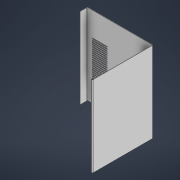
# Autodesk Inventor part: PlateAMP
Saved by Autodesk Inventor 2022 (Build 260153070, 153G)
## iProperties
Created: 2021-12-15
Part Number: PlateAMP
Material: Типовые
Document SubType Name: Sheet Metal
Designer: kalugin_a
Density: 1 g/cm^3
Flat Pattern Width: 26.5 cm
Flat Pattern Length: 43.9179 cm
Flat Pattern Area: 1163.82 cm^2
Sheet Metal Rule: По умолчанию_мм
Sheet Metal Width: 265,000 мм
Sheet Metal Length: 439,179 мм
Sheet Metal Area: 116382,371 мм^2
Appearance: По умолчанию
Author: kalugin_a
Autodesk Inventor part; units mm, degrees
ref_plane "YZ Plane" through (0, 0, 0) normal (1, 0, 0) x (0, 1, 0)
ref_plane "XZ Plane" through (0, 0, 0) normal (0, 1, 0) x (-1, 0, 0)
ref_plane "XY Plane" through (0, 0, 0) normal (0, 0, 1) x (1, 0, 0)
sketch "Эскиз1" plane through (0, 0, 0) normal (0, 0, 1) x (1, 0, 0)
  line L0 (0, 0) -> (217, 0)
  line L1 (217, 0) -> (217, 265)
  line L2 (217, 265) -> (0, 265)
  line L3 (0, 265) -> (0, 0)
  line L4 (207.9674, 23.6384) -> (147.9674, 23.6384) construction
  line L5 (206.4674, 25.1384) -> (149.4674, 25.1384)
  line L6 (149.4674, 22.1384) -> (206.4674, 22.1384)
  arc A0 (206.4674, 22.1384) -> (206.4674, 25.1384) centre (206.4674, 23.6384) ccw
  arc A1 (149.4674, 25.1384) -> (149.4674, 22.1384) centre (149.4674, 23.6384) ccw
  line L7 (207.9674, 29.6384) -> (147.9674, 29.6384) construction
  line L8 (206.4674, 31.1384) -> (149.4674, 31.1384)
  line L9 (149.4674, 28.1384) -> (206.4674, 28.1384)
  arc A2 (206.4674, 28.1384) -> (206.4674, 31.1384) centre (206.4674, 29.6384) ccw
  arc A3 (149.4674, 31.1384) -> (149.4674, 28.1384) centre (149.4674, 29.6384) ccw
  line L10 (207.9674, 35.6384) -> (147.9674, 35.6384) construction
  line L11 (206.4674, 37.1384) -> (149.4674, 37.1384)
  line L12 (149.4674, 34.1384) -> (206.4674, 34.1384)
  arc A4 (206.4674, 34.1384) -> (206.4674, 37.1384) centre (206.4674, 35.6384) ccw
  arc A5 (149.4674, 37.1384) -> (149.4674, 34.1384) centre (149.4674, 35.6384) ccw
  line L13 (207.9674, 41.6384) -> (147.9674, 41.6384) construction
  line L14 (206.4674, 43.1384) -> (149.4674, 43.1384)
  line L15 (149.4674, 40.1384) -> (206.4674, 40.1384)
  arc A6 (206.4674, 40.1384) -> (206.4674, 43.1384) centre (206.4674, 41.6384) ccw
  arc A7 (149.4674, 43.1384) -> (149.4674, 40.1384) centre (149.4674, 41.6384) ccw
  line L16 (207.9674, 47.6384) -> (147.9674, 47.6384) construction
  line L17 (206.4674, 49.1384) -> (149.4674, 49.1384)
  line L18 (149.4674, 46.1384) -> (206.4674, 46.1384)
  arc A8 (206.4674, 46.1384) -> (206.4674, 49.1384) centre (206.4674, 47.6384) ccw
  arc A9 (149.4674, 49.1384) -> (149.4674, 46.1384) centre (149.4674, 47.6384) ccw
  line L19 (207.9674, 53.6384) -> (147.9674, 53.6384) construction
  line L20 (206.4674, 55.1384) -> (149.4674, 55.1384)
  line L21 (149.4674, 52.1384) -> (206.4674, 52.1384)
  arc A10 (206.4674, 52.1384) -> (206.4674, 55.1384) centre (206.4674, 53.6384) ccw
  arc A11 (149.4674, 55.1384) -> (149.4674, 52.1384) centre (149.4674, 53.6384) ccw
  line L22 (207.9674, 59.6384) -> (147.9674, 59.6384) construction
  line L23 (206.4674, 61.1384) -> (149.4674, 61.1384)
  line L24 (149.4674, 58.1384) -> (206.4674, 58.1384)
  arc A12 (206.4674, 58.1384) -> (206.4674, 61.1384) centre (206.4674, 59.6384) ccw
  arc A13 (149.4674, 61.1384) -> (149.4674, 58.1384) centre (149.4674, 59.6384) ccw
  line L25 (207.9674, 65.6384) -> (147.9674, 65.6384) construction
  line L26 (206.4674, 67.1384) -> (149.4674, 67.1384)
  line L27 (149.4674, 64.1384) -> (206.4674, 64.1384)
  arc A14 (206.4674, 64.1384) -> (206.4674, 67.1384) centre (206.4674, 65.6384) ccw
  arc A15 (149.4674, 67.1384) -> (149.4674, 64.1384) centre (149.4674, 65.6384) ccw
  line L28 (207.9674, 71.6384) -> (147.9674, 71.6384) construction
  line L29 (206.4674, 73.1384) -> (149.4674, 73.1384)
  line L30 (149.4674, 70.1384) -> (206.4674, 70.1384)
  arc A16 (206.4674, 70.1384) -> (206.4674, 73.1384) centre (206.4674, 71.6384) ccw
  arc A17 (149.4674, 73.1384) -> (149.4674, 70.1384) centre (149.4674, 71.6384) ccw
  line L31 (207.9674, 77.6384) -> (147.9674, 77.6384) construction
  line L32 (206.4674, 79.1384) -> (149.4674, 79.1384)
  line L33 (149.4674, 76.1384) -> (206.4674, 76.1384)
  arc A18 (206.4674, 76.1384) -> (206.4674, 79.1384) centre (206.4674, 77.6384) ccw
  arc A19 (149.4674, 79.1384) -> (149.4674, 76.1384) centre (149.4674, 77.6384) ccw
  line L34 (207.9674, 83.6384) -> (147.9674, 83.6384) construction
  line L35 (206.4674, 85.1384) -> (149.4674, 85.1384)
  line L36 (149.4674, 82.1384) -> (206.4674, 82.1384)
  arc A20 (206.4674, 82.1384) -> (206.4674, 85.1384) centre (206.4674, 83.6384) ccw
  arc A21 (149.4674, 85.1384) -> (149.4674, 82.1384) centre (149.4674, 83.6384) ccw
  line L37 (207.9674, 89.6384) -> (147.9674, 89.6384) construction
  line L38 (206.4674, 91.1384) -> (149.4674, 91.1384)
  line L39 (149.4674, 88.1384) -> (206.4674, 88.1384)
  arc A22 (206.4674, 88.1384) -> (206.4674, 91.1384) centre (206.4674, 89.6384) ccw
  arc A23 (149.4674, 91.1384) -> (149.4674, 88.1384) centre (149.4674, 89.6384) ccw
  line L40 (207.9674, 95.6384) -> (147.9674, 95.6384) construction
  line L41 (206.4674, 97.1384) -> (149.4674, 97.1384)
  line L42 (149.4674, 94.1384) -> (206.4674, 94.1384)
  arc A24 (206.4674, 94.1384) -> (206.4674, 97.1384) centre (206.4674, 95.6384) ccw
  arc A25 (149.4674, 97.1384) -> (149.4674, 94.1384) centre (149.4674, 95.6384) ccw
  line L43 (207.9674, 101.6384) -> (147.9674, 101.6384) construction
  line L44 (206.4674, 103.1384) -> (149.4674, 103.1384)
  line L45 (149.4674, 100.1384) -> (206.4674, 100.1384)
  arc A26 (206.4674, 100.1384) -> (206.4674, 103.1384) centre (206.4674, 101.6384) ccw
  arc A27 (149.4674, 103.1384) -> (149.4674, 100.1384) centre (149.4674, 101.6384) ccw
  line L46 (207.9674, 107.6384) -> (147.9674, 107.6384) construction
  line L47 (206.4674, 109.1384) -> (149.4674, 109.1384)
  line L48 (149.4674, 106.1384) -> (206.4674, 106.1384)
  arc A28 (206.4674, 106.1384) -> (206.4674, 109.1384) centre (206.4674, 107.6384) ccw
  arc A29 (149.4674, 109.1384) -> (149.4674, 106.1384) centre (149.4674, 107.6384) ccw
  line L49 (207.9674, 113.6384) -> (147.9674, 113.6384) construction
  line L50 (206.4674, 115.1384) -> (149.4674, 115.1384)
  line L51 (149.4674, 112.1384) -> (206.4674, 112.1384)
  arc A30 (206.4674, 112.1384) -> (206.4674, 115.1384) centre (206.4674, 113.6384) ccw
  arc A31 (149.4674, 115.1384) -> (149.4674, 112.1384) centre (149.4674, 113.6384) ccw
  line L52 (207.9674, 119.6384) -> (147.9674, 119.6384) construction
  line L53 (206.4674, 121.1384) -> (149.4674, 121.1384)
  line L54 (149.4674, 118.1384) -> (206.4674, 118.1384)
  arc A32 (206.4674, 118.1384) -> (206.4674, 121.1384) centre (206.4674, 119.6384) ccw
  arc A33 (149.4674, 121.1384) -> (149.4674, 118.1384) centre (149.4674, 119.6384) ccw
  line L55 (207.9674, 125.6384) -> (147.9674, 125.6384) construction
  line L56 (206.4674, 127.1384) -> (149.4674, 127.1384)
  line L57 (149.4674, 124.1384) -> (206.4674, 124.1384)
  arc A34 (206.4674, 124.1384) -> (206.4674, 127.1384) centre (206.4674, 125.6384) ccw
  arc A35 (149.4674, 127.1384) -> (149.4674, 124.1384) centre (149.4674, 125.6384) ccw
  line L58 (207.9674, 131.6384) -> (147.9674, 131.6384) construction
  line L59 (206.4674, 133.1384) -> (149.4674, 133.1384)
  line L60 (149.4674, 130.1384) -> (206.4674, 130.1384)
  arc A36 (206.4674, 130.1384) -> (206.4674, 133.1384) centre (206.4674, 131.6384) ccw
  arc A37 (149.4674, 133.1384) -> (149.4674, 130.1384) centre (149.4674, 131.6384) ccw
  line L61 (207.9674, 137.6384) -> (147.9674, 137.6384) construction
  line L62 (206.4674, 139.1384) -> (149.4674, 139.1384)
  line L63 (149.4674, 136.1384) -> (206.4674, 136.1384)
  arc A38 (206.4674, 136.1384) -> (206.4674, 139.1384) centre (206.4674, 137.6384) ccw
  arc A39 (149.4674, 139.1384) -> (149.4674, 136.1384) centre (149.4674, 137.6384) ccw
  line L64 (207.9674, 143.6384) -> (147.9674, 143.6384) construction
  line L65 (206.4674, 145.1384) -> (149.4674, 145.1384)
  line L66 (149.4674, 142.1384) -> (206.4674, 142.1384)
  arc A40 (206.4674, 142.1384) -> (206.4674, 145.1384) centre (206.4674, 143.6384) ccw
  arc A41 (149.4674, 145.1384) -> (149.4674, 142.1384) centre (149.4674, 143.6384) ccw
  line L67 (207.9674, 149.6384) -> (147.9674, 149.6384) construction
  line L68 (206.4674, 151.1384) -> (149.4674, 151.1384)
  line L69 (149.4674, 148.1384) -> (206.4674, 148.1384)
  arc A42 (206.4674, 148.1384) -> (206.4674, 151.1384) centre (206.4674, 149.6384) ccw
  arc A43 (149.4674, 151.1384) -> (149.4674, 148.1384) centre (149.4674, 149.6384) ccw
  line L70 (207.9674, 155.6384) -> (147.9674, 155.6384) construction
  line L71 (206.4674, 157.1384) -> (149.4674, 157.1384)
  line L72 (149.4674, 154.1384) -> (206.4674, 154.1384)
  arc A44 (206.4674, 154.1384) -> (206.4674, 157.1384) centre (206.4674, 155.6384) ccw
  arc A45 (149.4674, 157.1384) -> (149.4674, 154.1384) centre (149.4674, 155.6384) ccw
  line L73 (207.9674, 161.6384) -> (147.9674, 161.6384) construction
  line L74 (206.4674, 163.1384) -> (149.4674, 163.1384)
  line L75 (149.4674, 160.1384) -> (206.4674, 160.1384)
  arc A46 (206.4674, 160.1384) -> (206.4674, 163.1384) centre (206.4674, 161.6384) ccw
  arc A47 (149.4674, 163.1384) -> (149.4674, 160.1384) centre (149.4674, 161.6384) ccw
  line L76 (77.9674, 23.6384) -> (17.9674, 23.6384) construction
  line L77 (76.4674, 25.1384) -> (19.4674, 25.1384)
  line L78 (19.4674, 22.1384) -> (76.4674, 22.1384)
  arc A48 (76.4674, 22.1384) -> (76.4674, 25.1384) centre (76.4674, 23.6384) ccw
  arc A49 (19.4674, 25.1384) -> (19.4674, 22.1384) centre (19.4674, 23.6384) ccw
  line L79 (77.9674, 29.6384) -> (17.9674, 29.6384) construction
  line L80 (76.4674, 31.1384) -> (19.4674, 31.1384)
  line L81 (19.4674, 28.1384) -> (76.4674, 28.1384)
  arc A50 (76.4674, 28.1384) -> (76.4674, 31.1384) centre (76.4674, 29.6384) ccw
  arc A51 (19.4674, 31.1384) -> (19.4674, 28.1384) centre (19.4674, 29.6384) ccw
  line L82 (77.9674, 35.6384) -> (17.9674, 35.6384) construction
  line L83 (76.4674, 37.1384) -> (19.4674, 37.1384)
  line L84 (19.4674, 34.1384) -> (76.4674, 34.1384)
  arc A52 (76.4674, 34.1384) -> (76.4674, 37.1384) centre (76.4674, 35.6384) ccw
  arc A53 (19.4674, 37.1384) -> (19.4674, 34.1384) centre (19.4674, 35.6384) ccw
  line L85 (77.9674, 41.6384) -> (17.9674, 41.6384) construction
  line L86 (76.4674, 43.1384) -> (19.4674, 43.1384)
  line L87 (19.4674, 40.1384) -> (76.4674, 40.1384)
  arc A54 (76.4674, 40.1384) -> (76.4674, 43.1384) centre (76.4674, 41.6384) ccw
  arc A55 (19.4674, 43.1384) -> (19.4674, 40.1384) centre (19.4674, 41.6384) ccw
  line L88 (77.9674, 47.6384) -> (17.9674, 47.6384) construction
  line L89 (76.4674, 49.1384) -> (19.4674, 49.1384)
  line L90 (19.4674, 46.1384) -> (76.4674, 46.1384)
  arc A56 (76.4674, 46.1384) -> (76.4674, 49.1384) centre (76.4674, 47.6384) ccw
  arc A57 (19.4674, 49.1384) -> (19.4674, 46.1384) centre (19.4674, 47.6384) ccw
  line L91 (77.9674, 53.6384) -> (17.9674, 53.6384) construction
  line L92 (76.4674, 55.1384) -> (19.4674, 55.1384)
  line L93 (19.4674, 52.1384) -> (76.4674, 52.1384)
  arc A58 (76.4674, 52.1384) -> (76.4674, 55.1384) centre (76.4674, 53.6384) ccw
  arc A59 (19.4674, 55.1384) -> (19.4674, 52.1384) centre (19.4674, 53.6384) ccw
  line L94 (77.9674, 59.6384) -> (17.9674, 59.6384) construction
  line L95 (76.4674, 61.1384) -> (19.4674, 61.1384)
  line L96 (19.4674, 58.1384) -> (76.4674, 58.1384)
  arc A60 (76.4674, 58.1384) -> (76.4674, 61.1384) centre (76.4674, 59.6384) ccw
  arc A61 (19.4674, 61.1384) -> (19.4674, 58.1384) centre (19.4674, 59.6384) ccw
  line L97 (77.9674, 65.6384) -> (17.9674, 65.6384) construction
  line L98 (76.4674, 67.1384) -> (19.4674, 67.1384)
  line L99 (19.4674, 64.1384) -> (76.4674, 64.1384)
  arc A62 (76.4674, 64.1384) -> (76.4674, 67.1384) centre (76.4674, 65.6384) ccw
  arc A63 (19.4674, 67.1384) -> (19.4674, 64.1384) centre (19.4674, 65.6384) ccw
  line L100 (77.9674, 71.6384) -> (17.9674, 71.6384) construction
  line L101 (76.4674, 73.1384) -> (19.4674, 73.1384)
  line L102 (19.4674, 70.1384) -> (76.4674, 70.1384)
  arc A64 (76.4674, 70.1384) -> (76.4674, 73.1384) centre (76.4674, 71.6384) ccw
  arc A65 (19.4674, 73.1384) -> (19.4674, 70.1384) centre (19.4674, 71.6384) ccw
  line L103 (77.9674, 77.6384) -> (17.9674, 77.6384) construction
  line L104 (76.4674, 79.1384) -> (19.4674, 79.1384)
  line L105 (19.4674, 76.1384) -> (76.4674, 76.1384)
  arc A66 (76.4674, 76.1384) -> (76.4674, 79.1384) centre (76.4674, 77.6384) ccw
  arc A67 (19.4674, 79.1384) -> (19.4674, 76.1384) centre (19.4674, 77.6384) ccw
  line L106 (77.9674, 83.6384) -> (17.9674, 83.6384) construction
  line L107 (76.4674, 85.1384) -> (19.4674, 85.1384)
  line L108 (19.4674, 82.1384) -> (76.4674, 82.1384)
  arc A68 (76.4674, 82.1384) -> (76.4674, 85.1384) centre (76.4674, 83.6384) ccw
  arc A69 (19.4674, 85.1384) -> (19.4674, 82.1384) centre (19.4674, 83.6384) ccw
  line L109 (77.9674, 89.6384) -> (17.9674, 89.6384) construction
  line L110 (76.4674, 91.1384) -> (19.4674, 91.1384)
  line L111 (19.4674, 88.1384) -> (76.4674, 88.1384)
  arc A70 (76.4674, 88.1384) -> (76.4674, 91.1384) centre (76.4674, 89.6384) ccw
  arc A71 (19.4674, 91.1384) -> (19.4674, 88.1384) centre (19.4674, 89.6384) ccw
  line L112 (77.9674, 95.6384) -> (17.9674, 95.6384) construction
  line L113 (76.4674, 97.1384) -> (19.4674, 97.1384)
  line L114 (19.4674, 94.1384) -> (76.4674, 94.1384)
  arc A72 (76.4674, 94.1384) -> (76.4674, 97.1384) centre (76.4674, 95.6384) ccw
  arc A73 (19.4674, 97.1384) -> (19.4674, 94.1384) centre (19.4674, 95.6384) ccw
  line L115 (77.9674, 101.6384) -> (17.9674, 101.6384) construction
  line L116 (76.4674, 103.1384) -> (19.4674, 103.1384)
  line L117 (19.4674, 100.1384) -> (76.4674, 100.1384)
  arc A74 (76.4674, 100.1384) -> (76.4674, 103.1384) centre (76.4674, 101.6384) ccw
  arc A75 (19.4674, 103.1384) -> (19.4674, 100.1384) centre (19.4674, 101.6384) ccw
  line L118 (77.9674, 107.6384) -> (17.9674, 107.6384) construction
  line L119 (76.4674, 109.1384) -> (19.4674, 109.1384)
  line L120 (19.4674, 106.1384) -> (76.4674, 106.1384)
  arc A76 (76.4674, 106.1384) -> (76.4674, 109.1384) centre (76.4674, 107.6384) ccw
  arc A77 (19.4674, 109.1384) -> (19.4674, 106.1384) centre (19.4674, 107.6384) ccw
  line L121 (77.9674, 113.6384) -> (17.9674, 113.6384) construction
  line L122 (76.4674, 115.1384) -> (19.4674, 115.1384)
  line L123 (19.4674, 112.1384) -> (76.4674, 112.1384)
  arc A78 (76.4674, 112.1384) -> (76.4674, 115.1384) centre (76.4674, 113.6384) ccw
  arc A79 (19.4674, 115.1384) -> (19.4674, 112.1384) centre (19.4674, 113.6384) ccw
  line L124 (77.9674, 119.6384) -> (17.9674, 119.6384) construction
  line L125 (76.4674, 121.1384) -> (19.4674, 121.1384)
  line L126 (19.4674, 118.1384) -> (76.4674, 118.1384)
  arc A80 (76.4674, 118.1384) -> (76.4674, 121.1384) centre (76.4674, 119.6384) ccw
  arc A81 (19.4674, 121.1384) -> (19.4674, 118.1384) centre (19.4674, 119.6384) ccw
  line L127 (77.9674, 125.6384) -> (17.9674, 125.6384) construction
  line L128 (76.4674, 127.1384) -> (19.4674, 127.1384)
  line L129 (19.4674, 124.1384) -> (76.4674, 124.1384)
  arc A82 (76.4674, 124.1384) -> (76.4674, 127.1384) centre (76.4674, 125.6384) ccw
  arc A83 (19.4674, 127.1384) -> (19.4674, 124.1384) centre (19.4674, 125.6384) ccw
  line L130 (77.9674, 131.6384) -> (17.9674, 131.6384) construction
  line L131 (76.4674, 133.1384) -> (19.4674, 133.1384)
  line L132 (19.4674, 130.1384) -> (76.4674, 130.1384)
  arc A84 (76.4674, 130.1384) -> (76.4674, 133.1384) centre (76.4674, 131.6384) ccw
  arc A85 (19.4674, 133.1384) -> (19.4674, 130.1384) centre (19.4674, 131.6384) ccw
  line L133 (77.9674, 137.6384) -> (17.9674, 137.6384) construction
  line L134 (76.4674, 139.1384) -> (19.4674, 139.1384)
  line L135 (19.4674, 136.1384) -> (76.4674, 136.1384)
  arc A86 (76.4674, 136.1384) -> (76.4674, 139.1384) centre (76.4674, 137.6384) ccw
  arc A87 (19.4674, 139.1384) -> (19.4674, 136.1384) centre (19.4674, 137.6384) ccw
  line L136 (77.9674, 143.6384) -> (17.9674, 143.6384) construction
  line L137 (76.4674, 145.1384) -> (19.4674, 145.1384)
  line L138 (19.4674, 142.1384) -> (76.4674, 142.1384)
  arc A88 (76.4674, 142.1384) -> (76.4674, 145.1384) centre (76.4674, 143.6384) ccw
  arc A89 (19.4674, 145.1384) -> (19.4674, 142.1384) centre (19.4674, 143.6384) ccw
  line L139 (77.9674, 149.6384) -> (17.9674, 149.6384) construction
  line L140 (76.4674, 151.1384) -> (19.4674, 151.1384)
  line L141 (19.4674, 148.1384) -> (76.4674, 148.1384)
  arc A90 (76.4674, 148.1384) -> (76.4674, 151.1384) centre (76.4674, 149.6384) ccw
  arc A91 (19.4674, 151.1384) -> (19.4674, 148.1384) centre (19.4674, 149.6384) ccw
  line L142 (77.9674, 155.6384) -> (17.9674, 155.6384) construction
  line L143 (76.4674, 157.1384) -> (19.4674, 157.1384)
  line L144 (19.4674, 154.1384) -> (76.4674, 154.1384)
  arc A92 (76.4674, 154.1384) -> (76.4674, 157.1384) centre (76.4674, 155.6384) ccw
  arc A93 (19.4674, 157.1384) -> (19.4674, 154.1384) centre (19.4674, 155.6384) ccw
  line L145 (77.9674, 161.6384) -> (17.9674, 161.6384) construction
  line L146 (76.4674, 163.1384) -> (19.4674, 163.1384)
  line L147 (19.4674, 160.1384) -> (76.4674, 160.1384)
  arc A94 (76.4674, 160.1384) -> (76.4674, 163.1384) centre (76.4674, 161.6384) ccw
  arc A95 (19.4674, 163.1384) -> (19.4674, 160.1384) centre (19.4674, 161.6384) ccw
  point P0 (177.9674, 23.6384)
  point P1 (177.9674, 29.6384)
  point P2 (177.9674, 35.6384)
  point P3 (177.9674, 41.6384)
  point P4 (177.9674, 47.6384)
  point P5 (177.9674, 53.6384)
  point P6 (177.9674, 59.6384)
  point P7 (177.9674, 65.6384)
  point P8 (177.9674, 71.6384)
  point P9 (177.9674, 77.6384)
  point P10 (177.9674, 83.6384)
  point P11 (177.9674, 89.6384)
  point P12 (177.9674, 95.6384)
  point P13 (177.9674, 101.6384)
  point P14 (177.9674, 107.6384)
  point P15 (177.9674, 113.6384)
  point P16 (177.9674, 119.6384)
  point P17 (177.9674, 125.6384)
  point P18 (177.9674, 131.6384)
  point P19 (177.9674, 137.6384)
  point P20 (177.9674, 143.6384)
  point P21 (177.9674, 149.6384)
  point P22 (177.9674, 155.6384)
  point P23 (177.9674, 161.6384)
  point P24 (47.9674, 23.6384)
  point P25 (47.9674, 29.6384)
  point P26 (47.9674, 35.6384)
  point P27 (47.9674, 41.6384)
  point P28 (47.9674, 47.6384)
  point P29 (47.9674, 53.6384)
  point P30 (47.9674, 59.6384)
  point P31 (47.9674, 65.6384)
  point P32 (47.9674, 71.6384)
  point P33 (47.9674, 77.6384)
  point P34 (47.9674, 83.6384)
  point P35 (47.9674, 89.6384)
  point P36 (47.9674, 95.6384)
  point P37 (47.9674, 101.6384)
  point P38 (47.9674, 107.6384)
  point P39 (47.9674, 113.6384)
  point P40 (47.9674, 119.6384)
  point P41 (47.9674, 125.6384)
  point P42 (47.9674, 131.6384)
  point P43 (47.9674, 137.6384)
  point P44 (47.9674, 143.6384)
  point P45 (47.9674, 149.6384)
  point P46 (47.9674, 155.6384)
  point P47 (47.9674, 161.6384)
  dimension "d11" = 265
  dimension "d12" = 217
  dimension "d33" = 60
  dimension "d34" = 3
  dimension "d50" = 6
  dimension "d53" = 130
  constraints: 392 end point, 288 point on circle, 96 centre point, 96 point on line, 4 tangent, 3 parallel, 2 horizontal, 2 perpendicular, 1 midpoint, 1 vertical, 658 other
  measures "d11" distance of L0.end L1.end
  measures "d12" distance of L1.end L2.end
  measures "d33" distance of L4.start L4.end
  measures "d34" diameter of A1
  measures "d50" distance of L5.start L8.start
  measures "d53" distance of L5.start L77.start
extrude "Пластина1" add sketch "Эскиз1" against normal blind 1.5 contours L3 L2 L1 L0 | A0 L6 A1 L5 | A2 L9 A3 L8 | A4 L12 A5 L11 | A6 L15 A7 L14 | A8 L18 A9 L17 | A10 L21 A11 L20 | A12 L24 A13 L23 | A14 L27 A15 L26 | A16 L30 A17 L29 | A18 L33 A19 L32 | A20 L36 A21 L35 | A22 L39 A23 L38 | A24 L42 A25 L41 | A26 L45 A27 L44 | A28 L48 A29 L47 | A30 L51 A31 L50 | A32 L54 A33 L53 | A34 L57 A35 L56 | A36 L60 A37 L59 | A38 L63 A39 L62 | A40 L66 A41 L65 | A42 L69 A43 L68 | A44 L72 A45 L71 | A46 L75 A47 L74 | A48 L78 A49 L77 | A50 L81 A51 L80 | A52 L84 A53 L83 | A54 L87 A55 L86 | A56 L90 A57 L89 | A58 L93 A59 L92 | A60 L96 A61 L95 | A62 L99 A63 L98 | A64 L102 A65 L101 | A66 L105 A67 L104 | A68 L108 A69 L107 | A70 L111 A71 L110 | A72 L114 A73 L113 | A74 L117 A75 L116 | A76 L120 A77 L119 | A78 L123 A79 L122 | A80 L126 A81 L125 | A82 L129 A83 L128 | A84 L132 A85 L131 | A86 L135 A87 L134 | A88 L138 A89 L137 | A90 L141 A91 L140 | A92 L144 A93 L143 | A94 L147 A95 L146
sketch "Эскиз2" plane through (1.5, 0, -1.5) normal (-1, 0, 0) x (0, -1, 0)
  line L0 (-265, 0) -> (0, 0)
  line L1 (0, 0) -> (0, 25)
  line L2 (0, 25) -> (-265, 25)
  line L3 (-265, 25) -> (-265, 0)
  constraints: 6 end point, 1 horizontal, 1 perpendicular, 1 vertical
edge flange "Фланец1" height 25 angle 90 thickness 1.5 bend radius 1.5 thickness toward (-1, 0, 0) relief straight relief width 1.5 relief depth 0.75 edges at (0, 132.5, 0) wall of the first edge with corners at (1.5, 265, -1.5) (1.5, 0, -1.5) (1.5, 0, 23.5) (1.5, 265, 23.5)
bend "Сгиб1"
corner "УглСтык1"
sketch "Эскиз3" plane through (215.5, 265, -1.5) normal (1, 0, 0) x (0, 1, 0)
  line L0 (-265, 0) -> (0, 0)
  line L1 (0, 0) -> (0, 200)
  line L2 (0, 200) -> (-265, 200)
  line L3 (-265, 200) -> (-265, 0)
  constraints: 6 end point, 1 horizontal, 1 perpendicular, 1 vertical
edge flange "Фланец2" height 200 angle 90 thickness 1.5 bend radius 1.5 thickness toward (1, 0, 0) relief straight relief width 1.5 relief depth 0.75 edges at (217, 132.5, 0) wall of the first edge with corners at (215.5, 0, -1.5) (215.5, 265, -1.5) (215.5, 265, 198.5) (215.5, 0, 198.5)
bend "Сгиб2"
corner "УглСтык2"
sketch "Эскиз4" plane through (217, 0, 197) normal (0, 0, 1) x (-1, 0, 0)
  line L0 (0, 265) -> (0, 0)
  line L1 (0, 0) -> (5, 0)
  line L2 (5, 0) -> (5, 265)
  line L3 (5, 265) -> (0, 265)
  constraints: 6 end point, 1 horizontal, 1 perpendicular, 1 vertical
edge flange "Фланец3" height 5 angle 90 thickness 1.5 bend radius 1.5 thickness toward (0, 0, 1) relief straight relief width 1.5 relief depth 0.75 edges at (217, 132.5, 198.5) wall of the first edge with corners at (217, 265, 197) (217, 0, 197) (212, 0, 197) (212, 265, 197)
bend "Сгиб3"
corner "УглСтык3"
sketch "Эскиз5" plane through (0, 0, -1.5) normal (0, 0, -1) x (-1, 0, 0)
  line L0 (-3, 317.8516) -> (-3, 52.8516)
  line L1 (-212, 317.8516) -> (-212, 52.8516)
  line L2 (-197, 185) -> (-147, 185) construction
  line L3 (-195.5, 183.5) -> (-148.5, 183.5)
  line L4 (-148.5, 186.5) -> (-195.5, 186.5)
  arc A0 (-195.5, 186.5) -> (-195.5, 183.5) centre (-195.5, 185) ccw
  arc A1 (-148.5, 183.5) -> (-148.5, 186.5) centre (-148.5, 185) ccw
  line L5 (-214, 265) -> (-3, 265) projected
  line L6 (-197, 179) -> (-147, 179) construction
  line L7 (-195.5, 177.5) -> (-148.5, 177.5)
  line L8 (-148.5, 180.5) -> (-195.5, 180.5)
  arc A2 (-195.5, 180.5) -> (-195.5, 177.5) centre (-195.5, 179) ccw
  arc A3 (-148.5, 177.5) -> (-148.5, 180.5) centre (-148.5, 179) ccw
  line L9 (-197, 173) -> (-147, 173) construction
  line L10 (-195.5, 171.5) -> (-148.5, 171.5)
  line L11 (-148.5, 174.5) -> (-195.5, 174.5)
  arc A4 (-195.5, 174.5) -> (-195.5, 171.5) centre (-195.5, 173) ccw
  arc A5 (-148.5, 171.5) -> (-148.5, 174.5) centre (-148.5, 173) ccw
  line L12 (-197, 167) -> (-147, 167) construction
  line L13 (-195.5, 165.5) -> (-148.5, 165.5)
  line L14 (-148.5, 168.5) -> (-195.5, 168.5)
  arc A6 (-195.5, 168.5) -> (-195.5, 165.5) centre (-195.5, 167) ccw
  arc A7 (-148.5, 165.5) -> (-148.5, 168.5) centre (-148.5, 167) ccw
  line L15 (-197, 161) -> (-147, 161) construction
  line L16 (-195.5, 159.5) -> (-148.5, 159.5)
  line L17 (-148.5, 162.5) -> (-195.5, 162.5)
  arc A8 (-195.5, 162.5) -> (-195.5, 159.5) centre (-195.5, 161) ccw
  arc A9 (-148.5, 159.5) -> (-148.5, 162.5) centre (-148.5, 161) ccw
  line L18 (-197, 155) -> (-147, 155) construction
  line L19 (-195.5, 153.5) -> (-148.5, 153.5)
  line L20 (-148.5, 156.5) -> (-195.5, 156.5)
  arc A10 (-195.5, 156.5) -> (-195.5, 153.5) centre (-195.5, 155) ccw
  arc A11 (-148.5, 153.5) -> (-148.5, 156.5) centre (-148.5, 155) ccw
  line L21 (-197, 149) -> (-147, 149) construction
  line L22 (-195.5, 147.5) -> (-148.5, 147.5)
  line L23 (-148.5, 150.5) -> (-195.5, 150.5)
  arc A12 (-195.5, 150.5) -> (-195.5, 147.5) centre (-195.5, 149) ccw
  arc A13 (-148.5, 147.5) -> (-148.5, 150.5) centre (-148.5, 149) ccw
  line L24 (-197, 143) -> (-147, 143) construction
  line L25 (-195.5, 141.5) -> (-148.5, 141.5)
  line L26 (-148.5, 144.5) -> (-195.5, 144.5)
  arc A14 (-195.5, 144.5) -> (-195.5, 141.5) centre (-195.5, 143) ccw
  arc A15 (-148.5, 141.5) -> (-148.5, 144.5) centre (-148.5, 143) ccw
  line L27 (-197, 137) -> (-147, 137) construction
  line L28 (-195.5, 135.5) -> (-148.5, 135.5)
  line L29 (-148.5, 138.5) -> (-195.5, 138.5)
  arc A16 (-195.5, 138.5) -> (-195.5, 135.5) centre (-195.5, 137) ccw
  arc A17 (-148.5, 135.5) -> (-148.5, 138.5) centre (-148.5, 137) ccw
  line L30 (-197, 131) -> (-147, 131) construction
  line L31 (-195.5, 129.5) -> (-148.5, 129.5)
  line L32 (-148.5, 132.5) -> (-195.5, 132.5)
  arc A18 (-195.5, 132.5) -> (-195.5, 129.5) centre (-195.5, 131) ccw
  arc A19 (-148.5, 129.5) -> (-148.5, 132.5) centre (-148.5, 131) ccw
  line L33 (-197, 125) -> (-147, 125) construction
  line L34 (-195.5, 123.5) -> (-148.5, 123.5)
  line L35 (-148.5, 126.5) -> (-195.5, 126.5)
  arc A20 (-195.5, 126.5) -> (-195.5, 123.5) centre (-195.5, 125) ccw
  arc A21 (-148.5, 123.5) -> (-148.5, 126.5) centre (-148.5, 125) ccw
  line L36 (-197, 119) -> (-147, 119) construction
  line L37 (-195.5, 117.5) -> (-148.5, 117.5)
  line L38 (-148.5, 120.5) -> (-195.5, 120.5)
  arc A22 (-195.5, 120.5) -> (-195.5, 117.5) centre (-195.5, 119) ccw
  arc A23 (-148.5, 117.5) -> (-148.5, 120.5) centre (-148.5, 119) ccw
  line L39 (-197, 113) -> (-147, 113) construction
  line L40 (-195.5, 111.5) -> (-148.5, 111.5)
  line L41 (-148.5, 114.5) -> (-195.5, 114.5)
  arc A24 (-195.5, 114.5) -> (-195.5, 111.5) centre (-195.5, 113) ccw
  arc A25 (-148.5, 111.5) -> (-148.5, 114.5) centre (-148.5, 113) ccw
  line L42 (-197, 107) -> (-147, 107) construction
  line L43 (-195.5, 105.5) -> (-148.5, 105.5)
  line L44 (-148.5, 108.5) -> (-195.5, 108.5)
  arc A26 (-195.5, 108.5) -> (-195.5, 105.5) centre (-195.5, 107) ccw
  arc A27 (-148.5, 105.5) -> (-148.5, 108.5) centre (-148.5, 107) ccw
  line L45 (-197, 101) -> (-147, 101) construction
  line L46 (-195.5, 99.5) -> (-148.5, 99.5)
  line L47 (-148.5, 102.5) -> (-195.5, 102.5)
  arc A28 (-195.5, 102.5) -> (-195.5, 99.5) centre (-195.5, 101) ccw
  arc A29 (-148.5, 99.5) -> (-148.5, 102.5) centre (-148.5, 101) ccw
  line L48 (-197, 95) -> (-147, 95) construction
  line L49 (-195.5, 93.5) -> (-148.5, 93.5)
  line L50 (-148.5, 96.5) -> (-195.5, 96.5)
  arc A30 (-195.5, 96.5) -> (-195.5, 93.5) centre (-195.5, 95) ccw
  arc A31 (-148.5, 93.5) -> (-148.5, 96.5) centre (-148.5, 95) ccw
  line L51 (-197, 89) -> (-147, 89) construction
  line L52 (-195.5, 87.5) -> (-148.5, 87.5)
  line L53 (-148.5, 90.5) -> (-195.5, 90.5)
  arc A32 (-195.5, 90.5) -> (-195.5, 87.5) centre (-195.5, 89) ccw
  arc A33 (-148.5, 87.5) -> (-148.5, 90.5) centre (-148.5, 89) ccw
  line L54 (-197, 83) -> (-147, 83) construction
  line L55 (-195.5, 81.5) -> (-148.5, 81.5)
  line L56 (-148.5, 84.5) -> (-195.5, 84.5)
  arc A34 (-195.5, 84.5) -> (-195.5, 81.5) centre (-195.5, 83) ccw
  arc A35 (-148.5, 81.5) -> (-148.5, 84.5) centre (-148.5, 83) ccw
  line L57 (-197, 77) -> (-147, 77) construction
  line L58 (-195.5, 75.5) -> (-148.5, 75.5)
  line L59 (-148.5, 78.5) -> (-195.5, 78.5)
  arc A36 (-195.5, 78.5) -> (-195.5, 75.5) centre (-195.5, 77) ccw
  arc A37 (-148.5, 75.5) -> (-148.5, 78.5) centre (-148.5, 77) ccw
  line L60 (-197, 71) -> (-147, 71) construction
  line L61 (-195.5, 69.5) -> (-148.5, 69.5)
  line L62 (-148.5, 72.5) -> (-195.5, 72.5)
  arc A38 (-195.5, 72.5) -> (-195.5, 69.5) centre (-195.5, 71) ccw
  arc A39 (-148.5, 69.5) -> (-148.5, 72.5) centre (-148.5, 71) ccw
  line L63 (-197, 65) -> (-147, 65) construction
  line L64 (-195.5, 63.5) -> (-148.5, 63.5)
  line L65 (-148.5, 66.5) -> (-195.5, 66.5)
  arc A40 (-195.5, 66.5) -> (-195.5, 63.5) centre (-195.5, 65) ccw
  arc A41 (-148.5, 63.5) -> (-148.5, 66.5) centre (-148.5, 65) ccw
  line L66 (-197, 59) -> (-147, 59) construction
  line L67 (-195.5, 57.5) -> (-148.5, 57.5)
  line L68 (-148.5, 60.5) -> (-195.5, 60.5)
  arc A42 (-195.5, 60.5) -> (-195.5, 57.5) centre (-195.5, 59) ccw
  arc A43 (-148.5, 57.5) -> (-148.5, 60.5) centre (-148.5, 59) ccw
  line L69 (-197, 53) -> (-147, 53) construction
  line L70 (-195.5, 51.5) -> (-148.5, 51.5)
  line L71 (-148.5, 54.5) -> (-195.5, 54.5)
  arc A44 (-195.5, 54.5) -> (-195.5, 51.5) centre (-195.5, 53) ccw
  arc A45 (-148.5, 51.5) -> (-148.5, 54.5) centre (-148.5, 53) ccw
  line L72 (-197, 47) -> (-147, 47) construction
  line L73 (-195.5, 45.5) -> (-148.5, 45.5)
  line L74 (-148.5, 48.5) -> (-195.5, 48.5)
  arc A46 (-195.5, 48.5) -> (-195.5, 45.5) centre (-195.5, 47) ccw
  arc A47 (-148.5, 45.5) -> (-148.5, 48.5) centre (-148.5, 47) ccw
  line L75 (-197, 41) -> (-147, 41) construction
  line L76 (-195.5, 39.5) -> (-148.5, 39.5)
  line L77 (-148.5, 42.5) -> (-195.5, 42.5)
  arc A48 (-195.5, 42.5) -> (-195.5, 39.5) centre (-195.5, 41) ccw
  arc A49 (-148.5, 39.5) -> (-148.5, 42.5) centre (-148.5, 41) ccw
  line L78 (-197, 35) -> (-147, 35) construction
  line L79 (-195.5, 33.5) -> (-148.5, 33.5)
  line L80 (-148.5, 36.5) -> (-195.5, 36.5)
  arc A50 (-195.5, 36.5) -> (-195.5, 33.5) centre (-195.5, 35) ccw
  arc A51 (-148.5, 33.5) -> (-148.5, 36.5) centre (-148.5, 35) ccw
  line L81 (-197, 29) -> (-147, 29) construction
  line L82 (-195.5, 27.5) -> (-148.5, 27.5)
  line L83 (-148.5, 30.5) -> (-195.5, 30.5)
  arc A52 (-195.5, 30.5) -> (-195.5, 27.5) centre (-195.5, 29) ccw
  arc A53 (-148.5, 27.5) -> (-148.5, 30.5) centre (-148.5, 29) ccw
  line L84 (-197, 23) -> (-147, 23) construction
  line L85 (-195.5, 21.5) -> (-148.5, 21.5)
  line L86 (-148.5, 24.5) -> (-195.5, 24.5)
  arc A54 (-195.5, 24.5) -> (-195.5, 21.5) centre (-195.5, 23) ccw
  arc A55 (-148.5, 21.5) -> (-148.5, 24.5) centre (-148.5, 23) ccw
  line L87 (-67, 185) -> (-17, 185) construction
  line L88 (-65.5, 183.5) -> (-18.5, 183.5)
  line L89 (-18.5, 186.5) -> (-65.5, 186.5)
  arc A56 (-65.5, 186.5) -> (-65.5, 183.5) centre (-65.5, 185) ccw
  arc A57 (-18.5, 183.5) -> (-18.5, 186.5) centre (-18.5, 185) ccw
  line L90 (-67, 179) -> (-17, 179) construction
  line L91 (-65.5, 177.5) -> (-18.5, 177.5)
  line L92 (-18.5, 180.5) -> (-65.5, 180.5)
  arc A58 (-65.5, 180.5) -> (-65.5, 177.5) centre (-65.5, 179) ccw
  arc A59 (-18.5, 177.5) -> (-18.5, 180.5) centre (-18.5, 179) ccw
  line L93 (-67, 173) -> (-17, 173) construction
  line L94 (-65.5, 171.5) -> (-18.5, 171.5)
  line L95 (-18.5, 174.5) -> (-65.5, 174.5)
  arc A60 (-65.5, 174.5) -> (-65.5, 171.5) centre (-65.5, 173) ccw
  arc A61 (-18.5, 171.5) -> (-18.5, 174.5) centre (-18.5, 173) ccw
  line L96 (-67, 167) -> (-17, 167) construction
  line L97 (-65.5, 165.5) -> (-18.5, 165.5)
  line L98 (-18.5, 168.5) -> (-65.5, 168.5)
  arc A62 (-65.5, 168.5) -> (-65.5, 165.5) centre (-65.5, 167) ccw
  arc A63 (-18.5, 165.5) -> (-18.5, 168.5) centre (-18.5, 167) ccw
  line L99 (-67, 161) -> (-17, 161) construction
  line L100 (-65.5, 159.5) -> (-18.5, 159.5)
  line L101 (-18.5, 162.5) -> (-65.5, 162.5)
  arc A64 (-65.5, 162.5) -> (-65.5, 159.5) centre (-65.5, 161) ccw
  arc A65 (-18.5, 159.5) -> (-18.5, 162.5) centre (-18.5, 161) ccw
  line L102 (-67, 155) -> (-17, 155) construction
  line L103 (-65.5, 153.5) -> (-18.5, 153.5)
  line L104 (-18.5, 156.5) -> (-65.5, 156.5)
  arc A66 (-65.5, 156.5) -> (-65.5, 153.5) centre (-65.5, 155) ccw
  arc A67 (-18.5, 153.5) -> (-18.5, 156.5) centre (-18.5, 155) ccw
  line L105 (-67, 149) -> (-17, 149) construction
  line L106 (-65.5, 147.5) -> (-18.5, 147.5)
  line L107 (-18.5, 150.5) -> (-65.5, 150.5)
  arc A68 (-65.5, 150.5) -> (-65.5, 147.5) centre (-65.5, 149) ccw
  arc A69 (-18.5, 147.5) -> (-18.5, 150.5) centre (-18.5, 149) ccw
  line L108 (-67, 143) -> (-17, 143) construction
  line L109 (-65.5, 141.5) -> (-18.5, 141.5)
  line L110 (-18.5, 144.5) -> (-65.5, 144.5)
  arc A70 (-65.5, 144.5) -> (-65.5, 141.5) centre (-65.5, 143) ccw
  arc A71 (-18.5, 141.5) -> (-18.5, 144.5) centre (-18.5, 143) ccw
  line L111 (-67, 137) -> (-17, 137) construction
  line L112 (-65.5, 135.5) -> (-18.5, 135.5)
  line L113 (-18.5, 138.5) -> (-65.5, 138.5)
  arc A72 (-65.5, 138.5) -> (-65.5, 135.5) centre (-65.5, 137) ccw
  arc A73 (-18.5, 135.5) -> (-18.5, 138.5) centre (-18.5, 137) ccw
  line L114 (-67, 131) -> (-17, 131) construction
  line L115 (-65.5, 129.5) -> (-18.5, 129.5)
  line L116 (-18.5, 132.5) -> (-65.5, 132.5)
  arc A74 (-65.5, 132.5) -> (-65.5, 129.5) centre (-65.5, 131) ccw
  arc A75 (-18.5, 129.5) -> (-18.5, 132.5) centre (-18.5, 131) ccw
  line L117 (-67, 125) -> (-17, 125) construction
  line L118 (-65.5, 123.5) -> (-18.5, 123.5)
  line L119 (-18.5, 126.5) -> (-65.5, 126.5)
  arc A76 (-65.5, 126.5) -> (-65.5, 123.5) centre (-65.5, 125) ccw
  arc A77 (-18.5, 123.5) -> (-18.5, 126.5) centre (-18.5, 125) ccw
  line L120 (-67, 119) -> (-17, 119) construction
  line L121 (-65.5, 117.5) -> (-18.5, 117.5)
  line L122 (-18.5, 120.5) -> (-65.5, 120.5)
  arc A78 (-65.5, 120.5) -> (-65.5, 117.5) centre (-65.5, 119) ccw
  arc A79 (-18.5, 117.5) -> (-18.5, 120.5) centre (-18.5, 119) ccw
  line L123 (-67, 113) -> (-17, 113) construction
  line L124 (-65.5, 111.5) -> (-18.5, 111.5)
  line L125 (-18.5, 114.5) -> (-65.5, 114.5)
  arc A80 (-65.5, 114.5) -> (-65.5, 111.5) centre (-65.5, 113) ccw
  arc A81 (-18.5, 111.5) -> (-18.5, 114.5) centre (-18.5, 113) ccw
  line L126 (-67, 107) -> (-17, 107) construction
  line L127 (-65.5, 105.5) -> (-18.5, 105.5)
  line L128 (-18.5, 108.5) -> (-65.5, 108.5)
  arc A82 (-65.5, 108.5) -> (-65.5, 105.5) centre (-65.5, 107) ccw
  arc A83 (-18.5, 105.5) -> (-18.5, 108.5) centre (-18.5, 107) ccw
  line L129 (-67, 101) -> (-17, 101) construction
  line L130 (-65.5, 99.5) -> (-18.5, 99.5)
  line L131 (-18.5, 102.5) -> (-65.5, 102.5)
  arc A84 (-65.5, 102.5) -> (-65.5, 99.5) centre (-65.5, 101) ccw
  arc A85 (-18.5, 99.5) -> (-18.5, 102.5) centre (-18.5, 101) ccw
  line L132 (-67, 95) -> (-17, 95) construction
  line L133 (-65.5, 93.5) -> (-18.5, 93.5)
  line L134 (-18.5, 96.5) -> (-65.5, 96.5)
  arc A86 (-65.5, 96.5) -> (-65.5, 93.5) centre (-65.5, 95) ccw
  arc A87 (-18.5, 93.5) -> (-18.5, 96.5) centre (-18.5, 95) ccw
  line L135 (-67, 89) -> (-17, 89) construction
  line L136 (-65.5, 87.5) -> (-18.5, 87.5)
  line L137 (-18.5, 90.5) -> (-65.5, 90.5)
  arc A88 (-65.5, 90.5) -> (-65.5, 87.5) centre (-65.5, 89) ccw
  arc A89 (-18.5, 87.5) -> (-18.5, 90.5) centre (-18.5, 89) ccw
  line L138 (-67, 83) -> (-17, 83) construction
  line L139 (-65.5, 81.5) -> (-18.5, 81.5)
  line L140 (-18.5, 84.5) -> (-65.5, 84.5)
  arc A90 (-65.5, 84.5) -> (-65.5, 81.5) centre (-65.5, 83) ccw
  arc A91 (-18.5, 81.5) -> (-18.5, 84.5) centre (-18.5, 83) ccw
  line L141 (-67, 77) -> (-17, 77) construction
  line L142 (-65.5, 75.5) -> (-18.5, 75.5)
  line L143 (-18.5, 78.5) -> (-65.5, 78.5)
  arc A92 (-65.5, 78.5) -> (-65.5, 75.5) centre (-65.5, 77) ccw
  arc A93 (-18.5, 75.5) -> (-18.5, 78.5) centre (-18.5, 77) ccw
  line L144 (-67, 71) -> (-17, 71) construction
  line L145 (-65.5, 69.5) -> (-18.5, 69.5)
  line L146 (-18.5, 72.5) -> (-65.5, 72.5)
  arc A94 (-65.5, 72.5) -> (-65.5, 69.5) centre (-65.5, 71) ccw
  arc A95 (-18.5, 69.5) -> (-18.5, 72.5) centre (-18.5, 71) ccw
  line L147 (-67, 65) -> (-17, 65) construction
  line L148 (-65.5, 63.5) -> (-18.5, 63.5)
  line L149 (-18.5, 66.5) -> (-65.5, 66.5)
  arc A96 (-65.5, 66.5) -> (-65.5, 63.5) centre (-65.5, 65) ccw
  arc A97 (-18.5, 63.5) -> (-18.5, 66.5) centre (-18.5, 65) ccw
  line L150 (-67, 59) -> (-17, 59) construction
  line L151 (-65.5, 57.5) -> (-18.5, 57.5)
  line L152 (-18.5, 60.5) -> (-65.5, 60.5)
  arc A98 (-65.5, 60.5) -> (-65.5, 57.5) centre (-65.5, 59) ccw
  arc A99 (-18.5, 57.5) -> (-18.5, 60.5) centre (-18.5, 59) ccw
  line L153 (-67, 53) -> (-17, 53) construction
  line L154 (-65.5, 51.5) -> (-18.5, 51.5)
  line L155 (-18.5, 54.5) -> (-65.5, 54.5)
  arc A100 (-65.5, 54.5) -> (-65.5, 51.5) centre (-65.5, 53) ccw
  arc A101 (-18.5, 51.5) -> (-18.5, 54.5) centre (-18.5, 53) ccw
  line L156 (-67, 47) -> (-17, 47) construction
  line L157 (-65.5, 45.5) -> (-18.5, 45.5)
  line L158 (-18.5, 48.5) -> (-65.5, 48.5)
  arc A102 (-65.5, 48.5) -> (-65.5, 45.5) centre (-65.5, 47) ccw
  arc A103 (-18.5, 45.5) -> (-18.5, 48.5) centre (-18.5, 47) ccw
  line L159 (-67, 41) -> (-17, 41) construction
  line L160 (-65.5, 39.5) -> (-18.5, 39.5)
  line L161 (-18.5, 42.5) -> (-65.5, 42.5)
  arc A104 (-65.5, 42.5) -> (-65.5, 39.5) centre (-65.5, 41) ccw
  arc A105 (-18.5, 39.5) -> (-18.5, 42.5) centre (-18.5, 41) ccw
  line L162 (-67, 35) -> (-17, 35) construction
  line L163 (-65.5, 33.5) -> (-18.5, 33.5)
  line L164 (-18.5, 36.5) -> (-65.5, 36.5)
  arc A106 (-65.5, 36.5) -> (-65.5, 33.5) centre (-65.5, 35) ccw
  arc A107 (-18.5, 33.5) -> (-18.5, 36.5) centre (-18.5, 35) ccw
  line L165 (-67, 29) -> (-17, 29) construction
  line L166 (-65.5, 27.5) -> (-18.5, 27.5)
  line L167 (-18.5, 30.5) -> (-65.5, 30.5)
  arc A108 (-65.5, 30.5) -> (-65.5, 27.5) centre (-65.5, 29) ccw
  arc A109 (-18.5, 27.5) -> (-18.5, 30.5) centre (-18.5, 29) ccw
  line L168 (-67, 23) -> (-17, 23) construction
  line L169 (-65.5, 21.5) -> (-18.5, 21.5)
  line L170 (-18.5, 24.5) -> (-65.5, 24.5)
  arc A110 (-65.5, 24.5) -> (-65.5, 21.5) centre (-65.5, 23) ccw
  arc A111 (-18.5, 21.5) -> (-18.5, 24.5) centre (-18.5, 23) ccw
  point P0 (0, 0)
  point P1 (-172, 185)
  point P2 (-172, 179)
  point P3 (-172, 173)
  point P4 (-172, 167)
  point P5 (-172, 161)
  point P6 (-172, 155)
  point P7 (-172, 149)
  point P8 (-172, 143)
  point P9 (-172, 137)
  point P10 (-172, 131)
  point P11 (-172, 125)
  point P12 (-172, 119)
  point P13 (-172, 113)
  point P14 (-172, 107)
  point P15 (-172, 101)
  point P16 (-172, 95)
  point P17 (-172, 89)
  point P18 (-172, 83)
  point P19 (-172, 77)
  point P20 (-172, 71)
  point P21 (-172, 65)
  point P22 (-172, 59)
  point P23 (-172, 53)
  point P24 (-172, 47)
  point P25 (-172, 41)
  point P26 (-172, 35)
  point P27 (-172, 29)
  point P28 (-172, 23)
  point P29 (-42, 185)
  point P30 (-42, 179)
  point P31 (-42, 173)
  point P32 (-42, 167)
  point P33 (-42, 161)
  point P34 (-42, 155)
  point P35 (-42, 149)
  point P36 (-42, 143)
  point P37 (-42, 137)
  point P38 (-42, 131)
  point P39 (-42, 125)
  point P40 (-42, 119)
  point P41 (-42, 113)
  point P42 (-42, 107)
  point P43 (-42, 101)
  point P44 (-42, 95)
  point P45 (-42, 89)
  point P46 (-42, 83)
  point P47 (-42, 77)
  point P48 (-42, 71)
  point P49 (-42, 65)
  point P50 (-42, 59)
  point P51 (-42, 53)
  point P52 (-42, 47)
  point P53 (-42, 41)
  point P54 (-42, 35)
  point P55 (-42, 29)
  point P56 (-42, 23)
  dimension "d35" = 50
  dimension "d36" = 3
  dimension "d56" = 80
  dimension "d57" = 15
  dimension "d60" = 6
  dimension "d63" = 130
  constraints: 452 end point, 336 point on circle, 112 centre point, 112 point on line, 4 tangent, 1 horizontal, 1 midpoint, 1 parallel, 1 vertical, 770 other
  measures "d35" distance of L2.start L2.end
  measures "d36" diameter of A1
  measures "d56" distance from line of L5 L2.end
  measures "d57" distance from line of L1 L2.start
  measures "d60" distance of L3.start L7.start
  measures "d63" distance of L3.start L88.start
extrude "Вырез1" cut sketch "Эскиз5" against normal blind 1.5
equation "\"d66\" = Толщина"
equation "\"d0\" = Толщина"
equation "\"d1\" = Ширина_просечки"
equation "\"d2\" = Глубина_просечки"
equation "\"d3\" = Мин_остаток"
equation "\"d4\" = Радиус_перехода"
equation "\"d7\" = Радиус_гибки"
equation "\"d8\" = Размер_просечки"
equation "\"d9\" = Размер_зазора"
equation "\"d10\" = Радиус_Якоби"
equation "\"d13\" = Ширина_просечки"
equation "\"d14\" = Глубина_просечки"
equation "\"d15\" = Мин_остаток"
equation "\"d16\" = Радиус_перехода"
equation "\"d19\" = Радиус_гибки"
equation "\"d20\" = Размер_просечки"
equation "\"d21\" = Размер_зазора"
equation "\"d22\" = Радиус_Якоби"
equation "\"d23\" = Ширина_просечки"
equation "\"d24\" = Глубина_просечки"
equation "\"d25\" = Мин_остаток"
equation "\"d26\" = Радиус_перехода"
equation "\"d29\" = Радиус_гибки"
equation "\"d30\" = Размер_просечки"
equation "\"d31\" = Размер_зазора"
equation "\"d32\" = Радиус_Якоби"
equation "\"Радиус_гибки\" = Толщина"
equation "\"Ширина_просечки\" = Толщина"
equation "\"Глубина_просечки\" = 0.5 * Толщина"
equation "\"Размер_просечки\" = 4 * Толщина"
equation "\"Мин_остаток\" = 2 * Толщина"
equation "\"Радиус_перехода\" = Радиус_гибки"
equation "\"Радиус_Якоби\" = Радиус_гибки"
equation "\"Размер_зазора\" = Толщина"
equation "\"Толщина\" = 1.5"
